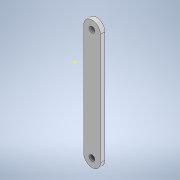
# Autodesk Inventor part: 2nd_part[1]
Saved by Autodesk Inventor 2022 (Build 260153000, 153)
## iProperties
Created: 2023-04-28
Part Number: 2nd_part[1]
Material: Generic
Document SubType Name: Modeling
Designer: Dell
Density: 1 g/cm^3
Appearance: Default
Author: Dell
Autodesk Inventor part; units mm, degrees
ref_plane "YZ Plane" through (0, 0, 0) normal (1, 0, 0) x (0, 1, 0)
ref_plane "XZ Plane" through (0, 0, 0) normal (0, 1, 0) x (-1, 0, 0)
ref_plane "XY Plane" through (0, 0, 0) normal (0, 0, 1) x (1, 0, 0)
sketch "Sketch1" plane through (0, 0, 0) normal (0, 0, 1) x (1, 0, 0)
  line L0 (15.2673, 33.0721) -> (15.2673, -66.9279) construction
  line L1 (7.7673, 33.0721) -> (7.7673, -66.9279)
  line L2 (22.7673, -66.9279) -> (22.7673, 33.0721)
  arc A0 (22.7673, 33.0721) -> (7.7673, 33.0721) centre (15.2673, 33.0721) ccw
  arc A1 (7.7673, -66.9279) -> (22.7673, -66.9279) centre (15.2673, -66.9279) ccw
  circle A2 centre (15.2673, 33.0721) radius 2.5
  circle A3 centre (15.2673, -66.9279) radius 2.5
  point P0 (0, 0)
  point P1 (15.2673, -16.9279)
  dimension "d0" = 100
  dimension "d1" = 15
  dimension "d2" = 5
  constraints: 8 end point, 4 centre point, 4 point on circle, 4 tangent, 2 coincident, 1 midpoint, 1 parallel, 1 vertical
  measures "d0" distance of L0.start L0.end
  measures "d1" diameter of A1
  measures "d2" diameter of A2
extrude "Extrusion1" add sketch "Sketch1" along normal blind 4
sketch "Sketch2" plane through (0, 0, 4) normal (0, 0, 1) x (1, 0, 0)
  point P0 (0, 0)
body "Solid1"
